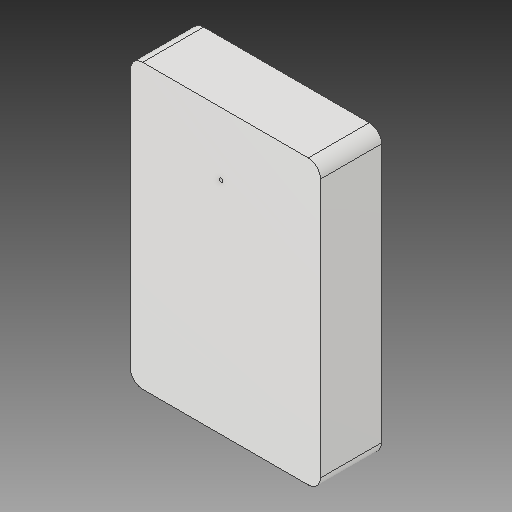
# Autodesk Inventor part: Ethernet switch
Saved by Autodesk Inventor 2017 (Build 210142000, 142)
## iProperties
Created: 2020-02-22
Part Number: Ethernet switch
Material: Acetal Resin, White
Document SubType Name: Modeling
Designer: S332848902
Density: 1.425 g/cm^3
Appearance: Smooth - White
Author: S332848902
Autodesk Inventor part; units mm, degrees
ref_plane "YZ Plane" through (0, 0, 0) normal (1, 0, 0) x (0, 1, 0)
ref_plane "XZ Plane" through (0, 0, 0) normal (0, 1, 0) x (-1, 0, 0)
ref_plane "XY Plane" through (0, 0, 0) normal (0, 0, 1) x (1, 0, 0)
sketch "Sketch1" plane through (0, 0, 0) normal (0, 0, 1) x (1, 0, 0)
  line L0 (0, 0) -> (69.215, 0)
  line L1 (69.215, 0) -> (69.215, -103.124)
  line L2 (69.215, -103.124) -> (0, -103.124)
  line L3 (0, -103.124) -> (0, 0)
  dimension "d0" = 69.215
  dimension "d1" = 103.124
  constraints: 8 end point, 2 parallel, 1 horizontal, 1 perpendicular
  measures "d0" distance of L1.end L2.end
  measures "d1" distance of L0.end L1.end
extrude "Extrusion1" add sketch "Sketch1" along normal blind 22.225
fillet "Fillet1" radius 4.445 3 edges at (0, 0, 11.1125) (69.215, 0, 11.1125) (0, -103.124, 11.1125)
fillet "Fillet2" radius 4.445 1 edges at (69.215, -103.124, 11.1125)
sketch "Sketch2" plane through (0, -98.679, 0) normal (-1, 0, 0) x (0, 0, 1)
  line L0 (0, 0) -> (0, 94.234) projected
  line L1 (22.225, 94.234) -> (0, 94.234) projected
  line L2 (0, 98.679) -> (22.225, 98.679) projected
  line L3 (5.461, 94.234) -> (18.161, 94.234)
  line L4 (18.161, 94.234) -> (18.161, 14.859)
  line L5 (18.161, 14.859) -> (5.461, 14.859)
  line L6 (5.461, 14.859) -> (5.461, 94.234)
  dimension "d8" = 12.7
  dimension "d9" = 79.375
  constraints: 8 end point, 2 parallel, 1 horizontal, 1 perpendicular, 1 point on line
  measures "d8" distance of L4.end L5.end
  measures "d9" distance of L3.end L4.end
extrude "Extrusion2" cut sketch "Sketch2" against normal blind 12.7
sketch "Sketch3" plane through (0, 0, 22.225) normal (0, 0, 1) x (1, 0, 0)
  line L0 (64.77, 0) -> (4.445, 0) projected
  circle A0 centre (33.02, -22.86) radius 0.635
  point P0 (0, 0)
  constraints: 1 centre point
extrude "Extrusion3" cut sketch "Sketch3" against normal blind 12.7
body "Solid1"
